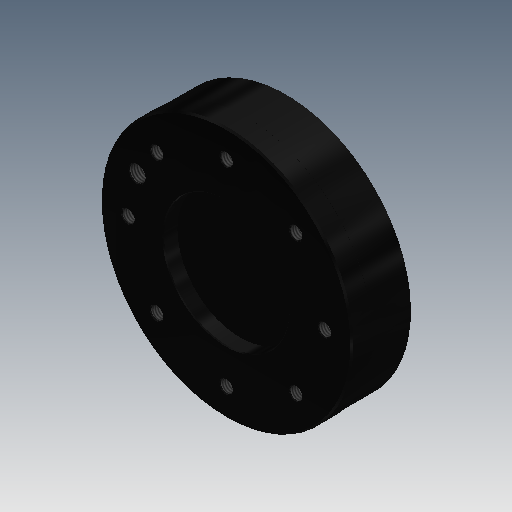
# Autodesk Inventor part: 210-100b
Saved by Autodesk Inventor 2020.1 (Build 241239000, 239)
## iProperties
Company: AUTODESK, INC.
Created: 2004-10-18
Part Number: 210-100b
Document SubType Name: Modeling
Designer: SCHNEIDER K.
Manufacturer: Standard
Standards Organization: Custom
Project: ADSK-000-000000
Description: FORE-ARM PIVOT HEAD MOUNING RING
Material: STEEL - HIGH GRADE ALLOY, BLACK OXIDE FINISH
Density: 1 g/cm^3
Appearance: Glossy - Black
Title: ROBOT
Author: SCHNEIDER K.
Revision Number: -
Autodesk Inventor part; units mm, degrees
ref_plane "YZ Plane" through (0, 0, 0) normal (1, 0, 0) x (0, 1, 0)
ref_plane "XZ Plane" through (0, 0, 0) normal (0, 1, 0) x (-1, 0, 0)
ref_plane "XY Plane" through (0, 0, 0) normal (0, 0, 1) x (1, 0, 0)
sketch "Sketch2" plane through (0, 0, 0) normal (1, 0, 0) x (0, 1, 0)
  line L0 (-80, 38) -> (0, 38)
  line L1 (-80, 38) -> (-80, 25.5)
  line L2 (-80, 25.5) -> (-79.5, 25)
  line L3 (-79.5, 25) -> (-79.5, 0)
  line L4 (-79.5, 0) -> (0, 0)
  line L5 (0, 38) -> (0, 0)
  line L6 (0, 0) -> (0, 10)
  constraints: 14 end point, 4 vertical, 2 horizontal
revolve "Revolve1" add sketch "Sketch2" angle 360 about axis through (0, 0, 0) along (0, 0, 1)
sketch "Sketch4" plane through (0, 0, 38) normal (0, 0, 1) x (1, 0, 0)
  circle A0 centre (0, 0) radius 80
  circle A1 centre (0, 0) radius 62.5 construction
  circle A2 centre (0, 0) radius 80 projected
  point P0 (0, 62.5)
  dimension "d12" = 125
  constraints: 2 coincident, 2 vertical alignment, 1 centre point, 2 other
hole "Hole2" at (0, 62.5, 38) direction (0, 0, -1) diameter 7.798 depth 25 tip angle 118 thread size "3/8-16 UNC" class "1B" standard "ANSI Unified Screw Threads"
pattern_circular "Circular Pattern1" count 8 over 360 about axis through (0, 0, 31.75) along (0, 0, 1) of "Hole2"
chamfer "Chamfer1" distance 1 angle 45 1 edges at (0, 80, 38)
sketch "Sketch3" plane through (0, 0, 38) normal (0, 0, 1) x (1, 0, 0)
  point P0 (0, 0)
hole "Hole1" at (0, 0, 38) direction (0, 0, -1) diameter 80 depth 9
chamfer "Chamfer2" distance 0.5 angle 45 9 edges at (-46.9512, 46.9512, 38) (-66.399, 0, 38) (-46.9512, -46.9512, 38) (0, -66.399, 38) (46.9512, -46.9512, 38) (66.399, 0, 38) (46.9512, 46.9512, 38) (0, 66.399, 38) (0, 40, 38)
sketch "Sketch5" plane through (0, 0, 38) normal (0, 0, 1) x (1, 0, 0)
  circle A0 centre (-44.1942, 44.1942) radius 4.399 projected
  circle A1 centre (0, 0) radius 40.5 projected
  circle A2 centre (0, 62.5) radius 4.399 projected
  circle A3 centre (-62.5, 0) radius 4.399 projected
  arc A4 (-44.1942, 44.1942) -> (-62.5, 0) centre (0, 0) ccw construction
  line L0 (0, 0) -> (0, 62.5) construction
  line L1 (0, 0) -> (-56.6442, 26.4136) construction
  dimension "d25" = 65
  constraints: 4 end point, 3 point on circle, 1 centre point, 1 coincident, 1 vertical
  measures "d25" angle of L0 L1
hole "Hole3" at (-56.6442, 26.4136, 38) direction (0, 0, -1) diameter 10.106 depth 15 tip angle 118 thread size "M12x1.75" class "6H" standard "ANSI Metric M Profile"
chamfer "Chamfer3" distance 0.5 angle 45 1 edges at (-56.6442, 31.4666, 38)
sketch "Sketch6" plane through (0, 0, 0) normal (0, 0, -1) x (-1, 0, 0)
  circle A0 centre (0, 0) radius 79.5 projected
  circle A1 centre (0, 0) radius 59.2292
  point P0 (-54.1926, 23.901)
  constraints: 1 coincident, 3 other
hole "Hole4" at (54.1926, 23.901, 0) direction (0, 0, 1) diameter 6.647 depth 12 tip angle 118 thread size "M8x1.25" class "6H" standard "ISO Metric profile"
pattern_circular "Circular Pattern2" count 8 over 360 about axis through (0, 0, 12.5) along (0, 0, 1) of "Hole4"
body "Solid1"
